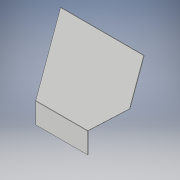
# Autodesk Inventor part: leftShoot
Saved by Autodesk Inventor 2017 (Build 210142000, 142)
## iProperties
Created: 2017-02-10
Part Number: leftShoot
Material: Generic
Document SubType Name: Sheet Metal
Designer: kingb
Density: 1 g/cm^3
Sheet Metal Rule: Default
Appearance: Default
Author: kingb
Autodesk Inventor part; units mm, degrees
ref_plane "YZ Plane" through (0, 0, 0) normal (1, 0, 0) x (0, 1, 0)
ref_plane "XZ Plane" through (0, 0, 0) normal (0, 1, 0) x (-1, 0, 0)
ref_plane "XY Plane" through (0, 0, 0) normal (0, 0, 1) x (1, 0, 0)
sketch "Sketch1" plane through (0, 0, 0) normal (0, 0, 1) x (1, 0, 0)
  line L0 (0, 0) -> (127, 0)
  line L1 (127, 0) -> (127, 50.8)
  line L2 (127, 50.8) -> (0, 50.8)
  line L3 (0, 50.8) -> (0, 0)
  dimension "d0" = 127
  dimension "d1" = 50.8
  measures "d0" distance of L2.end L1.end
  measures "d1" distance of L1.end L0.end
sketch "Sketch4" plane through (127, 217.3344, -60.7154) normal (0, -0.3420201, -0.9396926) x (-1, 0, 0)
  line L0 (127, 0) -> (0, 0)
  line L1 (0, 0) -> (-76.2, 0)
  line L2 (-76.2, 0) -> (-76.2, -101.6)
  line L3 (-76.2, -177.8) -> (0, -177.8) construction
  line L4 (0, -177.8) -> (0, 0)
  line L5 (0, -177.8) -> (-76.2, -101.6)
  line L6 (0, -177.8) -> (107.7631, -177.8) construction
  line L7 (-76.2, -101.6) -> (-76.2, -177.8) construction
  point P0 (127, -224.9934)
  dimension "d23" = 76.2
  dimension "d24" = 177.8
  dimension "d25" = 135
  measures "d23" distance of L3.end L3.start
  measures "d24" distance of L3.start L1.end
  measures "d25" angle of L6 L5
extrude "Plate1" add sketch "Sketch1" along normal blind 1.5875
sketch "Sketch3" plane through (127, 50.257, 0.0957) normal (0, 0.3420201, 0.9396926) x (-1, 0, 0)
  line L0 (127, 0) -> (0, 0)
  line L1 (0, 0) -> (0, -177.8)
  line L2 (0, -177.8) -> (127, -177.8)
  line L3 (127, -177.8) -> (127, 0)
  constraints: 6 end point, 1 horizontal, 1 perpendicular, 1 vertical
edge flange "Flange2" height 177.8 angle 20 thickness 1.5875 bend radius 1.5875 thickness toward (0, 0.3420201, 0.9396926) relief tear relief width 1.5875 relief depth 0.7937 edges at (63.5, 50.8, 0) wall of the first edge with corners at (0, 50.257, 0.0957) (127, 50.257, 0.0957) (127, 217.3344, -60.7154) (0, 217.3344, -60.7154)
bend "Bend2"
corner "Corner2"
sheet face with bend "Face2" sketch "Sketch4" thickness 1.5875 toward (0, 0.3420201, 0.9396926) bend radius 1.5875 relief tear relief width 1.5875 relief depth 0.7937
bend "Bend3"
equation "\"d13\" = BendReliefWidth"
equation "\"d14\" = BendReliefDepth"
equation "\"d15\" = MinimumRemnant"
equation "\"d16\" = BendRadius"
equation "\"d19\" = BendRadius"
equation "\"d20\" = CornerReliefSize"
equation "\"d21\" = GapSize"
equation "\"d22\" = JacobiRadiusSize"
equation "\"d26\" = BendRadius"
equation "\"d27\" = BendReliefWidth"
equation "\"d29\" = MinimumRemnant"
equation "\"d28\" = BendReliefDepth"
equation "\"d30\" = BendRadius"
equation "\"BendRadius\" = Thickness"
equation "\"BendReliefWidth\" = Thickness"
equation "\"BendReliefDepth\" = 0.5 * Thickness"
equation "\"CornerReliefSize\" = 4 * Thickness"
equation "\"MinimumRemnant\" = 2 * Thickness"
equation "\"TransitionRadius\" = BendRadius"
equation "\"JacobiRadiusSize\" = Thickness"
equation "\"GapSize\" = Thickness"
equation "\"d2\" = BendRadius"
equation "\"Thickness\" = 1.5875"
body "Solid1"
